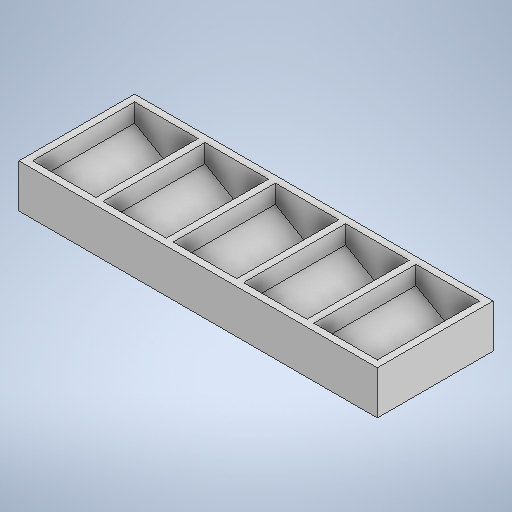
# Autodesk Inventor part: Bottom
Saved by Autodesk Inventor 2025 (Build 290162000, 162)
## iProperties
Created: 2024-08-06
Part Number: Bottom
Material: Generic
Document SubType Name: Modeling
Designer: ethan
Density: 1 g/cm^3
Appearance: Default
Author: ethan
Autodesk Inventor part; units mm, degrees
ref_plane "YZ Plane" through (0, 0, 0) normal (1, 0, 0) x (0, 1, 0)
ref_plane "XZ Plane" through (0, 0, 0) normal (0, 1, 0) x (-1, 0, 0)
sketch "Sketch1" plane through (0, 0, 0) normal (0, 0, 1) x (1, 0, 0)
  line L0 (17.78, -10.2653) -> (0, -20.5306)
  line L1 (0, -20.5306) -> (-17.78, -10.2653)
  line L2 (-17.78, -10.2653) -> (-17.78, 10.2653)
  line L3 (-17.78, 10.2653) -> (0, 20.5306)
  line L4 (0, 20.5306) -> (17.78, 10.2653)
  line L5 (17.78, 10.2653) -> (17.78, -10.2653)
  line L6 (0, 0) -> (20.8337, 0) construction
  line L7 (57.15, -10.2653) -> (39.37, -20.5306)
  line L8 (39.37, -20.5306) -> (21.59, -10.2653)
  line L9 (21.59, -10.2653) -> (21.59, 10.2653)
  line L10 (21.59, 10.2653) -> (39.37, 20.5306)
  line L11 (39.37, 20.5306) -> (57.15, 10.2653)
  line L12 (57.15, 10.2653) -> (57.15, -10.2653)
  line L13 (39.37, 0) -> (60.2037, 0) construction
  line L14 (96.52, -10.2653) -> (78.74, -20.5306)
  line L15 (78.74, -20.5306) -> (60.96, -10.2653)
  line L16 (60.96, -10.2653) -> (60.96, 10.2653)
  line L17 (60.96, 10.2653) -> (78.74, 20.5306)
  line L18 (78.74, 20.5306) -> (96.52, 10.2653)
  line L19 (96.52, 10.2653) -> (96.52, -10.2653)
  line L20 (78.74, 0) -> (99.5737, 0) construction
  line L21 (135.89, -10.2653) -> (118.11, -20.5306)
  line L22 (118.11, -20.5306) -> (100.33, -10.2653)
  line L23 (100.33, -10.2653) -> (100.33, 10.2653)
  line L24 (100.33, 10.2653) -> (118.11, 20.5306)
  line L25 (118.11, 20.5306) -> (135.89, 10.2653)
  line L26 (135.89, 10.2653) -> (135.89, -10.2653)
  line L27 (118.11, 0) -> (138.9437, 0) construction
  line L28 (175.26, -10.2653) -> (157.48, -20.5306)
  line L29 (157.48, -20.5306) -> (139.7, -10.2653)
  line L30 (139.7, -10.2653) -> (139.7, 10.2653)
  line L31 (139.7, 10.2653) -> (157.48, 20.5306)
  line L32 (157.48, 20.5306) -> (175.26, 10.2653)
  line L33 (175.26, 10.2653) -> (175.26, -10.2653)
  line L34 (157.48, 0) -> (178.3137, 0) construction
  line L35 (-17.78, 0) -> (-21.59, 0) construction
  line L36 (0, -20.5306) -> (0, -24.3406) construction
  line L37 (0, -24.3406) -> (-21.59, -24.3406) construction
  line L38 (-21.59, -24.3406) -> (-21.59, 0) construction
  line L39 (157.48, -20.5306) -> (157.48, -24.3406) construction
  line L40 (175.26, 0) -> (179.07, 0) construction
  line L41 (179.07, 0) -> (179.07, -24.3406) construction
  line L42 (179.07, -24.3406) -> (157.48, -24.3406) construction
  line L43 (-17.78, 0) -> (-21.59, 0)
  line L44 (-21.59, -24.3406) -> (-21.59, 0)
  line L45 (-21.59, -24.3406) -> (179.07, -24.3406)
  line L46 (179.07, -24.3406) -> (179.07, 0)
  line L47 (179.07, 0) -> (175.26, 0)
  line L48 (17.78, 0) -> (21.59, 0)
  line L49 (57.15, 0) -> (60.96, 0)
  line L50 (96.52, 0) -> (100.33, 0)
  line L51 (135.89, 0) -> (139.7, 0)
  dimension "d0" = 35.56
  dimension "d3" = 39.37
  dimension "d8" = 3.81
  dimension "d9" = 3.81
  dimension "d10" = 3.81
  dimension "d11" = 3.81
  constraints: 104 end point, 10 midpoint, 6 point on line, 5 coincident, 5 perpendicular, 4 horizontal, 3 vertical, 2 collinear, 76 other
  measures "d0" distance between parallel lines of L5 L2
  measures "d3" distance of point (0, 0) point (39.37, 0)
  measures "d8" distance of L35.start L35.end
  measures "d9" distance of L0.end L36.end
  measures "d10" distance of L28.end L39.end
  measures "d11" distance of L40.start L40.end
extrude "Extrusion1" add sketch "Sketch1" along normal blind 57.15 contours L5 L48 L9 L8 L7 L12 L49 L16 L15 L14 L19 L50 L23 L22 L21 L26 L51 L30 L29 L28 L33 L47 L46 L45 L44 L43 L2 L1 L0
sketch "Sketch2" plane through (0, 0, 57.15) normal (0, 0, 1) x (1, 0, 0)
  line L0 (-17.78, -10.2653) -> (-17.78, 0) construction
  line L1 (-17.78, 0) -> (-21.59, 0) construction
  line L2 (-21.59, 0) -> (-21.59, -24.3406) construction
  line L3 (-21.59, -24.3406) -> (179.07, -24.3406) construction
  line L4 (179.07, -24.3406) -> (179.07, 0) construction
  line L5 (179.07, 0) -> (175.26, 0) construction
  line L6 (175.26, 0) -> (175.26, -10.2653) construction
  line L7 (175.26, -10.2653) -> (157.48, -20.5306) construction
  line L8 (157.48, -20.5306) -> (139.7, -10.2653) construction
  line L9 (139.7, -10.2653) -> (139.7, 0) construction
  line L10 (139.7, 0) -> (135.89, 0) construction
  line L11 (135.89, 0) -> (135.89, -10.2653) construction
  line L12 (135.89, -10.2653) -> (118.11, -20.5306) construction
  line L13 (118.11, -20.5306) -> (100.33, -10.2653) construction
  line L14 (100.33, -10.2653) -> (100.33, 0) construction
  line L15 (100.33, 0) -> (96.52, 0) construction
  line L16 (96.52, 0) -> (96.52, -10.2653) construction
  line L17 (96.52, -10.2653) -> (78.74, -20.5306) construction
  line L18 (78.74, -20.5306) -> (60.96, -10.2653) construction
  line L19 (60.96, -10.2653) -> (60.96, 0) construction
  line L20 (60.96, 0) -> (57.15, 0) construction
  line L21 (57.15, 0) -> (57.15, -10.2653) construction
  line L22 (57.15, -10.2653) -> (39.37, -20.5306) construction
  line L23 (39.37, -20.5306) -> (21.59, -10.2653) construction
  line L24 (21.59, -10.2653) -> (21.59, 0) construction
  line L25 (21.59, 0) -> (17.78, 0) construction
  line L26 (17.78, 0) -> (17.78, -10.2653) construction
  line L27 (17.78, -10.2653) -> (0, -20.5306) construction
  line L28 (0, -20.5306) -> (-17.78, -10.2653) construction
  line L29 (-21.59, -24.3406) -> (179.07, -24.3406)
  line L30 (179.07, -24.3406) -> (179.07, 0)
  line L31 (179.07, 0) -> (-21.59, 0)
  line L32 (-21.59, 0) -> (-21.59, -24.3406)
  point P0 (0, 0)
  constraints: 8 end point, 2 parallel, 1 horizontal, 1 perpendicular
ref_plane "Work Plane1" through (0, 0, 28.575) normal (0, 0, 1) x (1, 0, 0)
extrude "Extrusion2" add sketch "Sketch2" along normal blind 3.81
mirror "Mirror1" about plane through (0, 0, 28.575) normal (0, 0, 1) of "Extrusion2"
body "Solid1"
